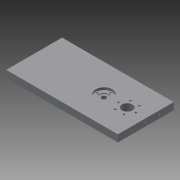
# Autodesk Inventor part: Traveler
Saved by Autodesk Inventor 2015 (Build 190159000, 159)
## iProperties
Created: 2015-01-23
Part Number: Traveler
Material: Generic
Document SubType Name: Modeling
Designer: chappelled
Density: 1 g/cm^3
Appearance: Default
Author: chappelled
Autodesk Inventor part; units mm, degrees
ref_plane "YZ Plane" through (0, 0, 0) normal (1, 0, 0) x (0, 1, 0)
ref_plane "XZ Plane" through (0, 0, 0) normal (0, 1, 0) x (-1, 0, 0)
ref_plane "XY Plane" through (0, 0, 0) normal (0, 0, 1) x (1, 0, 0)
sketch "Sketch1" plane through (0, 0, 0) normal (0, 1, 0) x (-1, 0, 0)
  line L0 (0, 0) -> (304.8, 0)
  line L1 (304.8, 0) -> (304.8, 152.4)
  line L2 (304.8, 152.4) -> (0, 152.4)
  line L3 (0, 152.4) -> (0, 0)
  dimension "d0" = 304.8
  dimension "d1" = 152.4
  constraints: 8 end point, 2 parallel, 1 horizontal, 1 perpendicular
  measures "d0" distance of L2.end L1.end
  measures "d1" distance of L1.end L0.end
extrude "Extrusion1" add sketch "Sketch1" along normal blind 12.7
hole "Hole1" at (-114.3, 12.7, 76.2) direction (0, -1, 0) diameter 12.7 end through all
hole "Hole2" at (-50.8, 12.7, 76.2) direction (0, -1, 0) diameter 28.575 end through all
hole "Hole3" at (-114.3, 0, 58.6994) direction (0, 1, 0) diameter 4.5 end through all countersink diameter 9.525 countersink angle 82
pattern_circular "Circular Pattern1" count 4 over 360 about axis through (-114.3, -328.3133, 76.2) along (0, 1, 0) of "Hole3"
sketch "Sketch4" plane through (0, 12.7, 0) normal (0, 1, 0) x (1, 0, 0)
  circle A0 centre (-114.3, -76.2) radius 6.35 projected
  circle A1 centre (-114.3, -76.2) radius 12.0332
  dimension "d41" = 24.0665
  constraints: 1 centre point, 1 coincident
  measures "d41" diameter of A1
sketch "Sketch5" plane through (0, 12.7, 0) normal (0, 1, 0) x (1, 0, 0)
  circle A0 centre (-50.8, -76.2) radius 14.2875 projected
  circle A1 centre (-114.3, -76.2) radius 6.35 projected
  line L0 (0, 0) -> (-304.8, 0) projected
  line L1 (-304.8, 0) -> (-304.8, -152.4) projected
  line L2 (-304.8, -152.4) -> (0, -152.4) projected
  line L3 (0, -152.4) -> (0, 0) projected
  circle A2 centre (-114.3, -76.2) radius 22.5425
  dimension "d42" = 45.085
  constraints: 1 centre point, 1 coincident
  measures "d42" diameter of A2
extrude "Extrusion4" add sketch "Sketch5" along normal blind 6.35 contours L3 L2 L1 L0
extrude "Extrusion5" cut sketch "Sketch4" against normal blind 2.032
hole "Hole4" at (-26.9748, 0, 76.2) direction (0, 1, 0) diameter 5.08 end through all countersink diameter 9.525 countersink angle 82
pattern_circular "Circular Pattern2" count 6 over 360 about axis through (-50.8, 19.05, 76.2) along (0, -1, 0) of "Hole4"
hole "Hole5" at (0, 9.525, 114.3) direction (-1, 0, 0) diameter 3.9624 depth 38.1 tip angle 118 thread size "10-32 UNF" class "2B" standard "ANSI Unified Screw Threads"
pattern_linear "Rectangular Pattern1" count 3 spacing 38.1 along (0, 0, -1) of "Hole5"
ref_plane "Work Plane1" through (-152.4, 0, 0) normal (-1, 0, 0) x (0, 0, 1)
mirror "Mirror1" about plane through (-152.4, 0, 0) normal (-1, 0, 0) of "Hole5", "Rectangular Pattern1"
body "Solid1"
